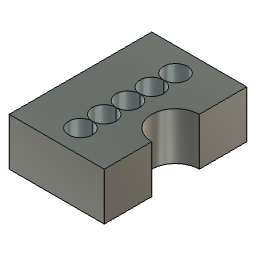
base_for_5_tips_press_fit (Autodesk Fusion 360 design; units mm, degrees)
Autodesk Fusion 360 part; units mm, degrees
sketch "Sketch1" plane through (0, 0, 0) normal (0, 0, 1) x (1, 0, 0)
  line L0 (-6.35, 9.525) -> (6.35, 9.525)
  line L1 (6.35, 9.525) -> (6.35, -9.525)
  line L2 (6.35, -9.525) -> (-6.35, -9.525)
  line L3 (-6.35, -9.525) -> (-6.35, 9.525)
  line L4 (0, 0) -> (0, 3.175) construction
  line L5 (0, 3.175) -> (0, 6.35) construction
  line L6 (0, 0) -> (0, -3.175) construction
  line L7 (0, -3.175) -> (0, -6.35) construction
  circle A0 centre (0, 6.35) radius 1.5875
  circle A1 centre (0, 3.175) radius 1.5875
  circle A2 centre (0, 0) radius 1.5875
  circle A3 centre (0, -3.175) radius 1.5875
  circle A4 centre (0, -6.35) radius 1.5875
  arc A5 (6.35, 3.175) -> (6.35, -3.175) centre (6.35, 0) ccw
  dimension "d3" = 12.7
  dimension "d4" = 19.05
  dimension "d5" = 3.175
  dimension "d6" = 3.175
  dimension "d7" = 3.175
  dimension "d8" = 3.175
  dimension "d9" = 3.175
  dimension "d10" = 3.175
  dimension "d11" = 3.175
  dimension "d12" = 3.175
  dimension "d13" = 3.175
  dimension "d21" = 6.35
  constraint horizontal L0
  constraint vertical L1
  constraint horizontal L2
  constraint vertical L3
  constraint coincident L4.start L6.start
  constraint vertical L4
  constraint parallel L4 L5
  constraint parallel L4 L6
  constraint parallel L6 L7
  constraint coincident L5.end A0.centre
  constraint coincident L4.end L5.start
  constraint coincident L6.end L7.start
  constraint coincident L7.end A4.centre
  constraint midpoint L1 A5.centre
  constraint coincident L1 A5.end
  constraint coincident L1 A5.start
  measures "d3" distance of L0.start L0.end
  measures "d4" distance of L0.start L2.end
  measures "d5" distance of L4.start L4.end
  measures "d6" distance of L4.end L5.end
  measures "d7" distance of L4.start L6.end
  measures "d8" distance of L6.end L7.end
  measures "d9" diameter of A0
  measures "d10" diameter of A1
  measures "d11" diameter of A2
  measures "d12" diameter of A3
  measures "d13" diameter of A4
  measures "d21" diameter of A5
extrude "Extrude1" add sketch "Sketch1" along normal blind 6.35 contours L0 L1 L2 L3 A5
sketch "Sketch2" plane through (0, 0, 6.35) normal (0, 0, 1) x (-1, 0, 0)
  circle A0 centre (0, 6.35) radius 1.5875
  circle A1 centre (0, -6.35) radius 1.5875
  line L0 (6.35, 9.525) -> (-6.35, 9.525)
  line L1 (-6.35, -3.175) -> (-6.35, -9.525)
  line L2 (-6.35, -9.525) -> (6.35, -9.525)
  line L3 (6.35, -9.525) -> (6.35, 9.525)
  arc A2 (1.905, 6.35) -> (-1.905, 6.35) centre (0, 6.35) ccw
  arc A3 (-1.905, -6.35) -> (1.905, -6.35) centre (0, -6.35) ccw
  circle A4 centre (0, -3.175) radius 1.5875
  arc A5 (0, -1.5875) -> (0, 1.5875) centre (0, 0) ccw
  arc A6 (0, 1.5875) -> (0, 4.7625) centre (0, 3.175) ccw
  arc A7 (0, -1.5875) -> (0, -4.7625) centre (0, -3.175) ccw
  arc A8 (0, 1.5875) -> (0, -1.5875) centre (0, 0) ccw
  arc A9 (0, 4.7625) -> (0, 1.5875) centre (0, 3.175) ccw
  line L4 (-6.35, 9.525) -> (-6.35, 3.175)
  arc A10 (-6.35, -3.175) -> (-6.35, 3.175) centre (-6.35, 0) ccw
  dimension "d17" = 3.81
  dimension "d18" = 3.81
  constraint concentric A0 A2
  constraint coincident L3 A2.start
  constraint concentric A1 A3
  measures "d17" diameter of A2
  measures "d18" diameter of A3
sketch "Sketch3" plane through (0, 0, 6.35) normal (0, 0, 1) x (-1, 0, 0)
  circle A0 centre (0, 6.35) radius 1.5875
  arc A1 (0, 1.5875) -> (0, 4.7625) centre (0, 3.175) ccw
  arc A2 (0, -1.5875) -> (0, 1.5875) centre (0, 0) ccw
  arc A3 (0, -4.7625) -> (0, -1.5875) centre (0, -3.175) ccw
  circle A4 centre (0, -6.35) radius 1.5875
  arc A5 (0, -1.5875) -> (0, -4.7625) centre (0, -3.175) ccw
  arc A6 (0, 1.5875) -> (0, -1.5875) centre (0, 0) ccw
  arc A7 (0, 4.7625) -> (0, 1.5875) centre (0, 3.175) ccw
  line L0 (-6.35, -3.175) -> (-6.35, -9.525)
  line L1 (-6.35, -9.525) -> (6.35, -9.525)
  line L2 (6.35, -9.525) -> (6.35, 9.525)
  line L3 (6.35, 9.525) -> (-6.35, 9.525)
  line L4 (-6.35, 9.525) -> (-6.35, 3.175)
  arc A8 (-6.35, -3.175) -> (-6.35, 3.175) centre (-6.35, 0) ccw
sketch "Sketch4" plane through (-6.35, 0, 0) normal (-1, 0, 0) x (0, -1, 0)
  line L0 (-9.525, 0) -> (9.525, 0)
  line L1 (9.525, 0) -> (9.525, 6.35)
  line L2 (9.525, 6.35) -> (-9.525, 6.35)
  line L3 (-9.525, 6.35) -> (-9.525, 0)
  line L4 (0, 0) -> (0, 3.175) construction
  circle A0 centre (0, 3.175) radius 1.905
  dimension "d22" = 3.175
  dimension "d23" = 3.81
  constraint coincident L4.start origin
  constraint perpendicular L0 L4
  constraint coincident L4.end A0.centre
  measures "d22" distance of L4.start L4.end
  measures "d23" diameter of A0
extrude "Extrude3" cut sketch "Sketch4" against normal blind 3.81 contours A0
thread "Thread1" "ANSI Unified Screw Threads 0.164(#8) 8-32 UNC 3B" major diameter 4.1656 minor diameter 3.4163 pitch 0.7937 angle 60 resizes the face on face at (-3.81, -1.8955, 2.9853)
equation "d9 = ( 1 / 8 ) * 1 in"
equation "d10 = ( 1 / 8 ) * 1 in"
equation "d11 = ( 1 / 8 ) * 1 in"
equation "d13 = ( 1 / 8 ) * 1 in"
equation "d21 = ( 1 / 4 ) * 1 in"
equation "d22 = ( 1 / 8 ) * 1 in"
